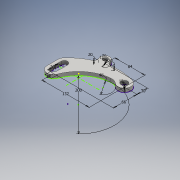
# Autodesk Inventor part: 스케치01
Saved by Autodesk Inventor 2016 (Build 200138000, 138)
## iProperties
Created: 2024-04-19
Part Number: 스케치01
Material: 일반
Document SubType Name: Modeling
Designer: pc
Density: 1 g/cm^3
Appearance: 기본값
Author: pc
Autodesk Inventor part; units mm, degrees
ref_plane "YZ Plane" through (0, 0, 0) normal (1, 0, 0) x (0, 1, 0)
ref_plane "XZ Plane" through (0, 0, 0) normal (0, 1, 0) x (-1, 0, 0)
ref_plane "XY Plane" through (0, 0, 0) normal (0, 0, 1) x (1, 0, 0)
sketch "스케치1" plane through (0, 0, 0) normal (0, 0, 1) x (1, 0, 0)
  line L0 (0, 33.6246) -> (0, -35.5266)
  line L1 (-57.2328, 0) -> (56.8423, 0)
  line L2 (-46.1794, 5.686) -> (-46.1794, -24.314) construction
  line L3 (-55.1794, 5.686) -> (-55.1794, -24.314)
  line L4 (-37.1794, -24.314) -> (-37.1794, 5.686)
  arc A0 (-37.1794, 5.686) -> (-55.1794, 5.686) centre (-46.1794, 5.686) ccw
  arc A1 (-55.1794, -24.314) -> (-37.1794, -24.314) centre (-46.1794, -24.314) ccw
  line L5 (-64.1794, 5.686) -> (-64.1794, -24.314)
  line L6 (-28.1794, 5.686) -> (-28.1794, -24.314)
  arc A2 (-56.1293, -9.314) -> (-55.1794, -9.9025) centre (-46.1794, 5.686) ccw
  arc A3 (-55.1794, -8.7256) -> (-56.1293, -9.314) centre (-46.1794, -24.314) ccw
  arc A4 (-37.1794, -9.9025) -> (-36.2296, -9.314) centre (-46.1794, 5.686) ccw
  arc A5 (-28.1794, 5.686) -> (-64.1794, 5.686) centre (-46.1794, 5.686) ccw
  arc A6 (-64.1794, -24.314) -> (-28.1794, -24.314) centre (-46.1794, -24.314) ccw
  arc A7 (-36.2296, -9.314) -> (-37.1794, -8.7256) centre (-46.1794, -24.314) ccw
  circle A8 centre (85.8206, 41.686) radius 9
  circle A9 centre (85.8206, 41.686) radius 18
  circle A10 centre (1.8206, 71.686) radius 6
  arc A11 (14.7648, 72.8891) -> (-9.5879, 65.4533) centre (1.8206, 71.686) ccw
  arc A12 (55.5566, 34.3887) -> (-29.295, -30.5524) centre (64.5072, -65.2099) ccw
  arc A13 (73.7709, 28.3141) -> (55.5566, 34.3887) centre (57.7047, 10.485) ccw
  arc A14 (91.2383, 58.8513) -> (-59.5617, 17.724) centre (47.7813, -78.8365) ccw
  arc A15 (-14.0792, 51.6232) -> (-9.5879, 65.4533) centre (-18.3636, 60.6589) ccw
  arc A16 (14.7648, 72.8891) -> (26.2155, 63.9268) centre (24.7219, 73.8146) ccw
  point P0 (0, 0)
  point P1 (-46.1794, -9.314)
  dimension "d0" = 18
  dimension "d2" = 30
  dimension "d5" = 18
  dimension "d6" = 36
  dimension "d7" = 132
  dimension "d8" = 66
  dimension "d9" = 12
  dimension "d10" = 26
  dimension "d11" = 84
  dimension "d12" = 30
  dimension "d13" = 200
  dimension "d15" = 48
  dimension "d16" = 20
  dimension "d17" = 20
  constraints: 34 point on circle, 17 centre point, 17 tangent, 16 end point, 4 coincident, 4 point on line, 2 vertical, 1 horizontal, 1 midpoint, 1 parallel, 1 other
  measures "d0" distance between parallel lines of L4 L3
  measures "d2" distance of L2.end L2.start
  measures "d5" diameter of A8
  measures "d6" diameter of A9
  measures "d7" horizontal distance of A8.centre L2.end
  measures "d8" vertical distance of A8.centre L2.end
  measures "d9" diameter of A10
  measures "d10" diameter of A11
  measures "d11" horizontal distance of A10.centre A8.centre
  measures "d12" vertical distance of A8.centre A10.centre
  measures "d13" diameter of A12
  measures "d15" diameter of A13
  measures "d16" diameter of A15
  measures "d17" diameter of A16
extrude "돌출1" add sketch "스케치1" along normal blind 10 contours A12 L1 L6 A5 A14 A9 A13 | A12 A6 L6 L1 | A9 | L6 A6 L5 A5 | A14 A15 A11 A16
sketch "스케치2" plane through (0, 0, 10) normal (0, 0, 1) x (1, 0, 0)
  point P0 (0, 0)
